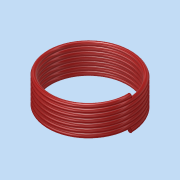
# Autodesk Inventor part: Coil
Saved by Autodesk Inventor 2017 (Build 210142000, 142)
## iProperties
Created: 2017-11-03
Part Number: Coil
Material: Copper, Alloy
Document SubType Name: Modeling
Designer: Derek Wider
Density: 8.92 g/cm^3
Appearance: Red
Author: Derek Wider
Autodesk Inventor part; units mm, degrees
ref_plane "YZ Plane" through (0, 0, 0) normal (1, 0, 0) x (0, 1, 0)
ref_plane "XZ Plane" through (0, 0, 0) normal (0, 1, 0) x (-1, 0, 0)
ref_plane "XY Plane" through (0, 0, 0) normal (0, 0, 1) x (1, 0, 0)
sketch "Sketch1" plane through (0, 0, 0) normal (0, 0, 1) x (1, 0, 0)
  circle A0 centre (12.065, 0) radius 0.635
  line L0 (0, 0) -> (0, 8.4359)
  dimension "d0" = 1.27
  dimension "d1" = 24.13
  constraints: 2 end point, 1 centre point, 1 vertical
  measures "d0" diameter of A0
  measures "d1" diameter of A0.centre L0
coil "Coil1" sketch "Sketch1" operation add axis through (0, 0, 0) along (0, 1, 0) pitch 1.2954 turns 7 hand right
body "Solid1"
